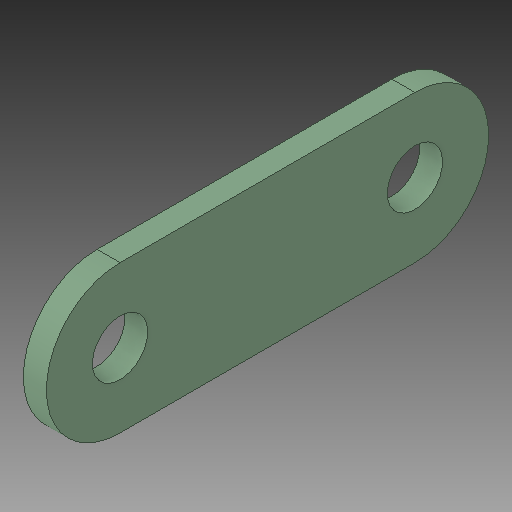
# Autodesk Inventor part: Part4
Saved by Autodesk Inventor 2019 (Build 230136000, 136)
## iProperties
Created: 2018-10-25
Part Number: Part4
Material: Iron, Gray
Document SubType Name: Modeling
Designer: Isaac
Density: 7.15 g/cm^3
Appearance: Rubber - Green
Mass: 11.7352 g
Surface Area: 16.9294 cm^2
Volume: 1.64128 cm^3
Author: Isaac
Autodesk Inventor part; units mm, degrees
ref_plane "YZ Plane" through (0, 0, 0) normal (1, 0, 0) x (0, 1, 0)
ref_plane "XZ Plane" through (0, 0, 0) normal (0, 1, 0) x (-1, 0, 0)
ref_plane "XY Plane" through (0, 0, 0) normal (0, 0, 1) x (1, 0, 0)
sketch "Sketch1" plane through (0, 0, 0) normal (1, 0, 0) x (0, 1, 0)
  line L0 (5.2977, -17.2418) -> (5.2977, 14.7582)
  arc A0 (5.2977, 14.7582) -> (-10.7023, 14.7582) centre (-2.7023, 14.7582) ccw
  line L1 (-10.7023, 14.7582) -> (-10.7023, -17.2418)
  arc A1 (-10.7023, -17.2418) -> (5.2977, -17.2418) centre (-2.7023, -17.2418) ccw
  circle A2 centre (-2.7023, 14.7582) radius 3
  circle A3 centre (-2.7023, -17.2418) radius 3
  point P0 (0, 0)
  dimension "d0" = 32
  dimension "d1" = 8
  dimension "d2" = 6
  constraints: 4 centre point, 4 end point, 4 point on circle, 4 tangent, 2 coincident, 2 equal radius, 1 vertical
  measures "d0" distance of L0.start L0.end
  measures "d1" radius of A0
  measures "d2" diameter of A2
extrude "Extrusion1" add sketch "Sketch1" along normal blind 2.5
body "Solid1"
